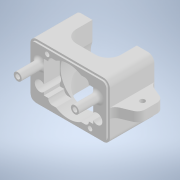
# Autodesk Inventor part: Housing_Vents
Saved by Autodesk Inventor 2021 (Build 250183000, 183)
## iProperties
Created: 2026-05-27
Part Number: Housing_Vents
Material: Generic
Document SubType Name: Modeling
Designer: Lukas
Density: 1 g/cm^3
Appearance: Default
Author: Lukas
Autodesk Inventor part; units mm, degrees
ref_plane "YZ Plane" through (0, 0, 0) normal (1, 0, 0) x (0, 1, 0)
ref_plane "XZ Plane" through (0, 0, 0) normal (0, 1, 0) x (-1, 0, 0)
ref_plane "XY Plane" through (0, 0, 0) normal (0, 0, 1) x (1, 0, 0)
sketch "Sketch1" plane through (0, 0, 0) normal (0, 0, 1) x (1, 0, 0)
  circle A0 centre (0, 0) radius 15
  circle A1 centre (-18, 6) radius 1.4
  circle A2 centre (-18, -6) radius 1.6
  circle A3 centre (18, -6) radius 1.6
  circle A4 centre (18, 6) radius 1.4
  line L0 (-21, 17.5) -> (21, 17.5)
  line L1 (25, 13.5) -> (25, -13.5)
  line L2 (21, -17.5) -> (-21, -17.5)
  line L3 (-25, -13.5) -> (-25, 13.5)
  arc A5 (-21, 17.5) -> (-25, 13.5) centre (-21, 13.5) ccw
  arc A6 (-25, -13.5) -> (-21, -17.5) centre (-21, -13.5) ccw
  arc A7 (21, -17.5) -> (25, -13.5) centre (21, -13.5) ccw
  arc A8 (25, 13.5) -> (21, 17.5) centre (21, 13.5) ccw
  point P0 (0, 17.5)
  point P1 (-25, 0)
  dimension "d0" = 36
  dimension "d1" = 12
  dimension "d2" = 6
  dimension "d3" = 18
  dimension "d4" = 2.8
  dimension "d5" = 30
  dimension "d6" = 35
  dimension "d7" = 50
  dimension "d8" = 4
  dimension "d30" = 3.2
  constraints: 9 centre point, 8 end point, 8 point on circle, 8 tangent, 5 equal radius, 3 horizontal alignment, 3 vertical alignment, 2 midpoint, 2 parallel, 1 coincident, 1 horizontal, 1 perpendicular
  measures "d0" distance of A4.centre A1.centre
  measures "d1" distance of A3.centre A4.centre
  measures "d2" vertical distance of point (0, 0) A3.centre
  measures "d3" horizontal distance of point (0, 0) A1.centre
  measures "d4" diameter of A1
  measures "d5" diameter of A0
  measures "d6" distance between parallel lines of L2 L0
  measures "d7" distance between parallel lines of L1 L3
  measures "d8" radius of A5
  measures "d30" diameter of A2
extrude "Extrusion1" add sketch "Sketch1" along normal blind 19
sketch "Sketch2" plane through (0, 0, 19) normal (0, 0, 1) x (1, 0, 0)
  line L0 (-21, -17.5) -> (21, -17.5) projected
  arc A0 (21, -17.5) -> (25, -13.5) centre (21, -13.5) ccw projected
  line L1 (25, -13.5) -> (25, 13.5) projected
  arc A1 (25, 13.5) -> (21, 17.5) centre (21, 13.5) ccw projected
  line L2 (21, 17.5) -> (-21, 17.5) projected
  arc A2 (-21, 17.5) -> (-25, 13.5) centre (-21, 13.5) ccw projected
  line L3 (-25, 13.5) -> (-25, -13.5) projected
  arc A3 (-25, -13.5) -> (-21, -17.5) centre (-21, -13.5) ccw projected
  circle A4 centre (0, 0) radius 15 projected
  circle A5 centre (-18, 6) radius 1.4 projected
  circle A6 centre (-18, -6) radius 1.6 projected
  circle A7 centre (18, -6) radius 1.6 projected
  circle A8 centre (18, 6) radius 1.4 projected
  line L4 (-10.25, 12.75) -> (10.25, 12.75)
  line L5 (12.75, 10.25) -> (12.75, -10.25)
  line L6 (10.25, -12.75) -> (-10.25, -12.75)
  line L7 (-12.75, -10.25) -> (-12.75, 10.25)
  arc A9 (-10.25, 12.75) -> (-12.75, 10.25) centre (-10.25, 10.25) ccw
  arc A10 (12.75, 10.25) -> (10.25, 12.75) centre (10.25, 10.25) ccw
  arc A11 (10.25, -12.75) -> (12.75, -10.25) centre (10.25, -10.25) ccw
  arc A12 (-12.75, -10.25) -> (-10.25, -12.75) centre (-10.25, -10.25) ccw
  line L8 (-15.5, 10) -> (15.5, 10)
  line L9 (15.5, 10) -> (15.5, -10)
  line L10 (15.5, -10) -> (-15.5, -10)
  line L11 (-15.5, -10) -> (-15.5, 10)
  circle A13 centre (-13.5, 13.5) radius 1.4
  circle A14 centre (13.5, -13.5) radius 1.4
  point P0 (0, 12.75)
  point P1 (-12.75, 0)
  point P2 (-7.9017, 12.75)
  point P3 (7.9017, 12.75)
  point P4 (12.75, 7.9017)
  point P5 (12.75, -7.9017)
  point P6 (7.9017, -12.75)
  point P7 (-7.9017, -12.75)
  point P8 (-12.75, -7.9017)
  point P9 (-12.75, 7.9017)
  point P10 (-15.5, 0)
  point P11 (0, 10)
  point P12 (12.75, 10)
  point P13 (12.75, -10)
  point P14 (-12.75, -10)
  point P15 (-12.75, 10)
  dimension "d11" = 2.5
  dimension "d12" = 25.5
  dimension "d15" = 31
  dimension "d16" = 20
  dimension "d17" = 13.5
  dimension "d18" = 13.5
  dimension "d19" = 13.5
  dimension "d20" = 13.5
  dimension "d21" = 2.8
  constraints: 16 end point, 8 point on circle, 8 tangent, 6 centre point, 4 equal radius, 4 midpoint, 4 parallel, 3 perpendicular, 2 horizontal, 2 horizontal alignment, 2 vertical alignment
  measures "d11" radius of A9
  measures "d12" distance between parallel lines of L5 L7
  measures "d15" distance of L8.start L8.end
  measures "d16" distance of L8.end L9.end
  measures "d17" horizontal distance of point (0, 0) A13.centre
  measures "d18" horizontal distance of A14.centre point (0, 0)
  measures "d19" horizontal distance of A13.centre point (0, 0)
  measures "d20" horizontal distance of A14.centre point (0, 0)
  measures "d21" diameter of A13
extrude "Extrusion2" add sketch "Sketch2" along normal blind 10
sketch "Sketch3" plane through (0, 0, 29) normal (0, 0, 1) x (1, 0, 0)
  circle A0 centre (-18, -6) radius 1.6 projected
  circle A1 centre (-18, -6) radius 1.6 projected
  circle A2 centre (18, -6) radius 1.6 projected
  circle A3 centre (18, -6) radius 1.6 projected
  circle A4 centre (-18, -6) radius 3.25
  circle A5 centre (18, -6) radius 1.6 projected
  circle A6 centre (18, -6) radius 3.25
  point P0 (0, 0)
  dimension "d23" = 6.5
  constraints: 2 centre point, 2 coincident, 1 equal radius
  measures "d23" diameter of A6
extrude "Extrusion3" cut sketch "Sketch3" against normal blind 27 contours A0 | A2 | A4 | A6
sketch "Sketch8" plane through (0, 0, 29) normal (0, 0, 1) x (1, 0, 0)
  line L0 (21, 17.5) -> (-21, 17.5) projected
  arc A0 (-21, 17.5) -> (-25, 13.5) centre (-21, 13.5) ccw projected
  line L1 (-25, 13.5) -> (-25, -13.5) projected
  arc A1 (-25, -13.5) -> (-21, -17.5) centre (-21, -13.5) ccw projected
  line L2 (-21, -17.5) -> (21, -17.5) projected
  arc A2 (21, -17.5) -> (25, -13.5) centre (21, -13.5) ccw projected
  line L3 (25, -13.5) -> (25, 13.5) projected
  arc A3 (25, 13.5) -> (21, 17.5) centre (21, 13.5) ccw projected
  line L4 (-21, 16.3) -> (21, 16.3)
  arc A4 (23.8, 13.5) -> (21, 16.3) centre (21, 13.5) ccw
  line L5 (23.8, 13.5) -> (23.8, -13.5)
  arc A5 (21, -16.3) -> (23.8, -13.5) centre (21, -13.5) ccw
  line L6 (21, -16.3) -> (-21, -16.3)
  arc A6 (-23.8, -13.5) -> (-21, -16.3) centre (-21, -13.5) ccw
  line L7 (-23.8, -13.5) -> (-23.8, 13.5)
  arc A7 (-21, 16.3) -> (-23.8, 13.5) centre (-21, 13.5) ccw
  point P0 (0, 0)
  dimension "d48" = 1.2
  constraints: 8 end point, 8 point on circle, 4 centre point, 7 other
  measures "d48" distance between parallel lines of L0 L4
extrude "Extrusion8" cut sketch "Sketch8" against normal blind 1
sketch "Sketch4" plane through (0, 0, 29) normal (0, 0, 1) x (1, 0, 0)
  circle A0 centre (-18, 6) radius 1.4 projected
  circle A1 centre (-18, 6) radius 2.5
  circle A2 centre (18, 6) radius 1.4 projected
  circle A3 centre (18, 6) radius 2.5
  point P0 (0, 0)
  dimension "d26" = 5
  constraints: 2 centre point, 2 coincident, 1 equal radius
  measures "d26" diameter of A1
extrude "Extrusion4" add sketch "Sketch4" along normal blind 14
fillet "Fillet1" radius 2 3 edges at (18, 3.5, 29) (18, 8.5, 29) (-20.5, 6, 29)
sketch "Sketch5" plane through (0, 0, 0) normal (0, 1, 0) x (-1, 0, 0)
  line L0 (-25, 0) -> (-25, 28) projected
  line L1 (-25, 0) -> (-25, 28) projected
  line L2 (-25, 26) -> (-37, 21)
  line L3 (-37, 21) -> (-37, 7)
  line L4 (-37, 7) -> (-25, 2)
  circle A0 centre (-31.5, 14) radius 1.6
  point P0 (0, 0)
  point P1 (-37, 14)
  point P2 (-25, 14)
  point P3 (-25, 2)
  point P4 (-25, 26)
  dimension "d31" = 14
  dimension "d32" = 5
  dimension "d33" = 12
  dimension "d52" = 5.5
  dimension "d53" = 3.2
  constraints: 6 end point, 2 horizontal alignment, 2 midpoint, 2 point on line, 1 centre point, 1 equal length, 1 vertical
  measures "d31" distance of L2.end L3.end
  measures "d32" vertical distance of L2.start L2.end
  measures "d33" horizontal distance of L2.start L2.end
  measures "d52" distance from line of L3 A0.centre
  measures "d53" diameter of A0
extrude "Extrusion5" add sketch "Sketch5" along normal mid plane 6
sketch "Sketch6" plane through (-21, -17.5, 0) normal (0, -1, 0) x (1, 0, 0)
  line L0 (36, 19) -> (36, 0) projected
  line L1 (6, 19) -> (6, 0) projected
  line L2 (6, 19) -> (13.0983, 19) projected
  line L3 (28.9017, 19) -> (36, 19) projected
  line L4 (0, 0) -> (42, 0) projected
  line L5 (7, 18) -> (35, 18)
  line L6 (35, 18) -> (35, 0)
  line L7 (35, 0) -> (7, 0)
  line L8 (7, 0) -> (7, 18)
  point P0 (21, 0)
  point P1 (21, 18)
  point P2 (21, 0)
  point P3 (7, 0)
  dimension "d36" = 28
  dimension "d37" = 18
  constraints: 8 end point, 2 midpoint, 2 parallel, 1 horizontal, 1 perpendicular, 1 point on line, 1 vertical alignment
  measures "d36" distance of L5.start L5.end
  measures "d37" distance of L5.end L6.end
extrude "Extrusion6" cut sketch "Sketch6" against normal through all
fillet "Fillet2" radius 8 4 edges at (14, 11.4426, 18) (14, -11.4426, 18) (-14, -11.4426, 18) (-14, 11.4426, 18)
fillet "Fillet4" radius 5 4 edges at (25, 0, 2) (37, 0, 7) (37, 0, 21) (25, 0, 26)
equation "\"d2\" = 0.5 * d1"
equation "\"d3\" = 0.5 * d0"
equation "\"d18\" = d17"
equation "\"d20\" = d19"
body "Solid1"
